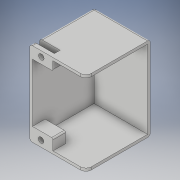
# Autodesk Inventor part: Caixa KS
Saved by Autodesk Inventor 2019 (Build 230136000, 136)
## iProperties
Created: 2022-03-20
Part Number: Caixa KS
Material: Genérico
Document SubType Name: Modeling
Designer: Hanter
Density: 1 g/cm^3
Appearance: Padrão
Author: Hanter
Autodesk Inventor part; units mm, degrees
ref_plane "YZ Plane" through (0, 0, 0) normal (1, 0, 0) x (0, 1, 0)
ref_plane "XZ Plane" through (0, 0, 0) normal (0, 1, 0) x (-1, 0, 0)
ref_plane "XY Plane" through (0, 0, 0) normal (0, 0, 1) x (1, 0, 0)
sketch "Esboço1" plane through (0, 0, 0) normal (0, 1, 0) x (-1, 0, 0)
  line L0 (-20.5, 23.5) -> (20.5, 23.5)
  line L1 (20.5, 23.5) -> (20.5, -23.5)
  line L2 (20.5, -23.5) -> (-20.5, -23.5)
  line L3 (-20.5, -23.5) -> (-20.5, 23.5)
  line L4 (-20.5, 23.5) -> (20.5, -23.5) construction
  line L5 (20.5, 23.5) -> (-20.5, -23.5) construction
  point P0 (0, 0)
  dimension "d0" = 41
  dimension "d1" = 47
  constraints: 12 end point, 2 midpoint, 2 parallel, 1 horizontal, 1 perpendicular
  measures "d0" distance of L1.end L2.end
  measures "d1" distance of L0.end L1.end
extrude "Extrusão1" add sketch "Esboço1" along normal blind 61
shell "Casca1" thickness 2 removed faces 2 at (6.8333, 20.3333, 23.5) at (20.5, 20.3333, -7.8333)
sketch "Esboço4" plane through (-20.5, 0, 23.5) normal (0, 0, 1) x (1, 0, 0)
  line L0 (2, 2) -> (2, 59) projected
  line L1 (2, 59) -> (15, 59)
  line L2 (15, 59) -> (15, 54.5)
  line L3 (15, 54.5) -> (2, 54.5)
  line L4 (2, 54.5) -> (2, 59)
  line L5 (41, 2) -> (2, 2) projected
  line L6 (2, 2) -> (15, 2)
  line L7 (15, 2) -> (15, 7.5)
  line L8 (15, 7.5) -> (2, 7.5)
  line L9 (2, 7.5) -> (2, 2)
  arc A0 (7.6282, 59) -> (9.3718, 59) centre (8.5, 57.2) ccw
  circle A1 centre (8.3, 4.5) radius 2
  line L10 (41, 0) -> (0, 0) projected
  line L11 (0, 0) -> (0, 61) projected
  line L12 (0, 61) -> (41, 61) projected
  point P0 (20.5, 0)
  dimension "d15" = 13
  dimension "d16" = 4.5
  dimension "d17" = 13
  dimension "d18" = 5.5
  dimension "d19" = 4
  dimension "d20" = 4
  dimension "d21" = 4.5
  dimension "d22" = 8.3
  dimension "d23" = 3.8
  dimension "d24" = 8.5
  constraints: 16 end point, 4 parallel, 2 centre point, 2 horizontal, 2 perpendicular, 2 point on circle, 2 point on line
  measures "d15" distance of L2.end L3.end
  measures "d16" distance of L1.end L2.end
  measures "d17" distance of L8.end L7.end
  measures "d18" distance of L7.end L6.end
  measures "d19" diameter of A0
  measures "d20" diameter of A1
  measures "d21" distance from line of L10 A1.centre
  measures "d22" distance from line of L11 A1.centre
  measures "d23" distance from line of L12 A0.centre
  measures "d24" distance from line of L11 A0.centre
extrude "Extrusão2" add sketch "Esboço4" against normal blind 3 contours L0 L1 A0 L2 L3 | L0 L8 L7 L5
fillet "Arredondamento4" radius 4 2 edges at (20.5, 60, 23.5) (20.5, 1, 23.5)
sketch "Esboço11" plane through (-18.5, 2, -21.5) normal (1, 0, 0) x (0, 0, -1)
  line L0 (-42, 5.5) -> (-42, 0) projected
  line L1 (-45, -2) -> (2, -2) projected
  line L2 (-42, 5.5) -> (-37.8, 5.5)
  line L3 (-37.8, 5.5) -> (-37.8, -2)
  line L4 (-37.8, -2) -> (-42, -2)
  line L5 (-42, -2) -> (-42, 5.5)
  line L6 (-42, 57) -> (-42, 52.5) projected
  line L7 (-42, 52.5) -> (-37.8, 52.5)
  line L8 (-37.8, 52.5) -> (-37.8, 59.7447)
  line L9 (-37.8, 59.7447) -> (-42, 59.7447)
  line L10 (-42, 59.7447) -> (-42, 52.5)
  point P0 (-21.5, -2)
  dimension "d47" = 4.2
  dimension "d48" = 4.2
  constraints: 16 end point, 4 parallel, 2 horizontal, 2 perpendicular, 1 point on line
  measures "d47" distance of L3.end L4.end
  measures "d48" distance of L9.end L8.end
extrude "Extrusão8" cut sketch "Esboço11" along normal blind 13 and the other way blind 2
sketch "Esboço12" plane through (-18.5, 2, -21.5) normal (1, 0, 0) x (0, 0, -1)
  line L0 (-37.8, -2) -> (-37.8, 0) projected
  line L1 (-37.8, -2) -> (-35.8, -2)
  line L2 (-35.8, -2) -> (-35.8, 8)
  line L3 (-35.8, 8) -> (-37.8, 8)
  line L4 (-37.8, 8) -> (-37.8, -2)
  line L5 (-45, 5.5) -> (-42, 5.5) projected
  line L6 (-45, 5.5) -> (-37.8, 5.5)
  line L7 (-37.8, 5.5) -> (-37.8, 8)
  line L8 (-37.8, 8) -> (-45, 8)
  line L9 (-45, 8) -> (-45, 5.5)
  line L10 (-45, 52.5) -> (-42, 52.5) projected
  line L11 (-45, 52.5) -> (-35.8, 52.5)
  line L12 (-35.8, 52.5) -> (-35.8, 50.5)
  line L13 (-35.8, 50.5) -> (-45, 50.5)
  line L14 (-45, 50.5) -> (-45, 52.5)
  line L15 (-37.8, 59) -> (-42, 59) projected
  line L16 (-35.8, 52.5) -> (-37.8, 52.5)
  line L17 (-37.8, 52.5) -> (-37.8, 59)
  line L18 (-37.8, 59) -> (-35.8, 59)
  line L19 (-35.8, 59) -> (-35.8, 52.5)
  point P0 (-21.5, -2)
  dimension "d53" = 2
  dimension "d54" = 10
  dimension "d55" = 9.2
  dimension "d56" = 2
  constraints: 32 end point, 8 parallel, 4 horizontal, 4 perpendicular
  measures "d53" distance of L3.end L2.end
  measures "d54" distance of L2.end L1.end
  measures "d55" distance of L12.end L13.end
  measures "d56" distance of L11.end L12.end
extrude "Extrusão9" add sketch "Esboço12" along normal blind 13
sketch "Esboço13" plane through (-5.5, 54.5, 16.3) normal (1, 0, 0) x (0, 0, -1)
  line L0 (2, -44.5) -> (-7.2, -44.5) projected
  line L1 (2, -52.5) -> (2, -44.5) projected
  line L2 (-7.2, -44.5) -> (2, -44.5)
  line L3 (2, -44.5) -> (2, -52.5)
  line L4 (2, -52.5) -> (-7.2, -52.5)
  line L5 (-7.2, -52.5) -> (-7.2, -44.5)
  line L6 (-7.2, -2) -> (2, -2) projected
  line L7 (-3.2, 4.5) -> (37.8, 4.5) projected
  line L8 (-7.2, -2) -> (2, -2)
  line L9 (2, -2) -> (2, 4.5)
  line L10 (2, 4.5) -> (-7.2, 4.5)
  line L11 (-7.2, 4.5) -> (-7.2, -2)
  point P0 (16.3, -54.5)
  constraints: 16 end point, 4 parallel, 2 horizontal, 2 perpendicular, 2 point on line
extrude "Extrusão10" add sketch "Esboço13" along normal blind 2
fillet "Arredondamento5" radius 2 2 edges at (-20.5, 61, 22) (-20.5, 0, 22)
fillet "Arredondamento6" radius 2 2 edges at (-20.5, 61, -3.6) (-20.5, 0, -3.6)
fillet "Arredondamento7" radius 2 5 edges at (-19.9142, 60.4142, -23.5) (1, 61, -23.5) (-19.9142, 0.5858, -23.5) (1, 0, -23.5) (-20.5, 30.5, -23.5)
fillet "Arredondamento10" radius 1 2 edges at (-3.5, 52.5, 18.9) (-3.5, 10, 18.9)
